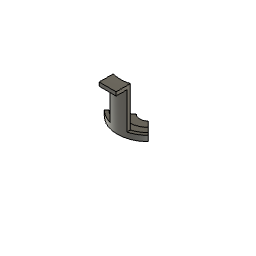
Wafer Loader 2 (Autodesk Fusion 360 design; units mm, degrees)
Autodesk Fusion 360 part; units mm, degrees
sketch "Sketch1" plane through (0, 0, 0) normal (0, 0, 1) x (1, 0, 0)
  circle A0 centre (0, 0) radius 51.3
  circle A1 centre (0, 0) radius 76
  circle A2 centre (0, 0) radius 23.25
  line L0 (0, 0) -> (-54.6679, -54.6679)
  line L1 (0, 0) -> (75, 0) construction
  line L2 (0, 0) -> (0, -76)
  line L3 (0, 0) -> (54.6679, -54.6679)
  line L4 (0, 0) -> (-23.1763, -71.3292)
  line L5 (0, 0) -> (75, 0) construction
  line L6 (0, 0) -> (23.1763, -71.3292)
  line L7 (-23.1763, -71.3292) -> (23.1763, -71.3292)
  line L8 (-23.1763, -71.3292) -> (-23.1763, -81.3292)
  line L9 (23.1763, -71.3292) -> (23.1763, -81.3292)
  line L10 (-23.1763, -81.3292) -> (23.1763, -81.3292)
  line L11 (-23.1763, -81.3292) -> (-23.1763, -111.3292)
  line L12 (23.1763, -81.3292) -> (23.1763, -111.3292)
  line L13 (-23.1763, -111.3292) -> (23.1763, -111.3292)
  circle A3 centre (0, 0) radius 85
  line L14 (-53.7401, -53.7401) -> (-60.1041, -60.1041)
  line L15 (53.7401, -53.7401) -> (60.1041, -60.1041)
  line L16 (-23.1763, -111.3292) -> (-23.1763, -101.3292)
  line L17 (-23.1763, -101.3292) -> (23.1763, -101.3292)
  dimension "d1" = 102.6
  dimension "d2" = 152
  dimension "d3" = 46.5
  dimension "d4" = 135
  dimension "d5" = 108
  dimension "d6" = 10
  dimension "d7" = 30
  dimension "d12" = 170
  dimension "d15" = 10
  constraint coincident A0.centre A1.centre
  constraint concentric A0 A1
  constraint horizontal L1
  constraint coincident A1 L2.end
  constraint vertical L2
  constraint symmetric A0.centre L2 A1.centre
  constraint symmetric L0.end L2 L3.end
  constraint horizontal L5
  constraint symmetric L2 A0.centre A1.centre
  constraint symmetric L2 L4.end L6.end
  constraint perpendicular L7 L8
  constraint symmetric L2 L8.end L9.end
  constraint perpendicular L10 L11
  constraint symmetric L2 L11.end L12.end
  constraint concentric A1 A3
  constraint coincident A1 L14.start
  constraint coincident L0 L14.start
  constraint coincident A3 L14.end
  constraint parallel L0 L14
  constraint coincident A1 L15.start
  constraint coincident L3 L15.start
  constraint coincident A3 L15.end
  constraint parallel L3 L15
  constraint perpendicular L13 L16
  constraint coincident L12 L17.end
  constraint perpendicular L12 L17
  measures "d1" diameter of A0
  measures "d2" diameter of A1
  measures "d3" diameter of A2
  measures "d4" angle of L0 L1
  measures "d5" angle of L4 L5
  measures "d6" distance of L4.end L8.end
  measures "d7" distance of L8.end L11.end
  measures "d12" diameter of A3
  measures "d15" distance of L11.end L16.end
extrude "Extrude1" add sketch "Sketch1" along normal blind 5 contours A0 A2 L0 L4 | A0 A1 L0 L4 L8 | A0 A1 L3 L6 L9 | A0 A2 L3 L6 | A0 A2 L2 L4 | A0 L2 L4 L7 | A0 L2 L6 L7 | A0 A2 L2 L6 | A1 L2 L7 L8 | A1 L2 L7 L9
extrude "Extrude2" add sketch "Sketch1" along normal blind 10 contours A0 A1 L0 L4 L8 | A0 A1 L3 L6 L9 | A0 L2 L4 L7 | A0 L2 L6 L7 | A1 L2 L7 L8 | A1 L2 L7 L9
extrude "Extrude3" add sketch "Sketch1" along normal blind 15 contours A1 L0 L3 A3 L14 L15 | A1 L0 L8 L11 A3 L14 | A1 L3 L9 L12 A3 L15 | A1 L8 L9 L10 | L10 L11 L12 A3
extrude "Extrude4" add sketch "Sketch1" along normal blind 15 contours L10 L11 L12 A3 | L11 L12 A3 L17 | L11 L12 L13 L16 L17
revolve "Revolve1" add 1 faces at (47.9183, -47.9183, 5) angle 45 about axis through (0, 0, -221.3292) along (0, 0, 1)
revolve "Revolve2" add 1 faces at (-47.9183, -47.9183, 5) angle 45 about axis through (0, 0, -221.3292) along (0, 0, -1)
extrude "Extrude5" cut sketch "Sketch1" along normal blind 15 contours L11 L12 L13 L16 L17
extrude "Extrude6" cut sketch "Sketch1" along normal blind 10 contours A1 L8 L9 L10 | L10 L11 L12 A3 | L11 L12 A3 L17
extrude "Extrude7" add 1 faces at (0, -92.8862, 10) along direction (0, 0, -1) blind 10
extrude "Extrude8" cut sketch "Sketch1" along normal blind 15 contours A0 A2 L0 L3 | A0 A1 L0 L3 | A1 L0 L3 A3 L14 L15
extrude "Extrude9" add sketch "Sketch1" along normal blind 100 contours A1 L8 L9 L10
extrude "Extrude10" cut sketch "Sketch1" along normal blind 100 contours L10 L11 L12 A3 | L11 L12 A3 L17
extrude "Extrude11" add sketch "Sketch1" along normal blind 100 contours L10 L11 L12 A3 | L11 L12 A3 L17 | L11 L12 L13 L16 L17
extrude "Extrude12" cut sketch "Sketch1" along normal blind 92 contours L10 L11 L12 A3 | L11 L12 A3 L17 | L11 L12 L13 L16 L17
extrude "Extrude13" add sketch "Sketch1" along normal blind 92 contours L10 L11 L12 A3
extrude "Extrude14" cut sketch "Sketch1" along normal blind 100 contours L11 L12 A3 L17 | L11 L12 L13 L16 L17
extrude "Extrude15" add 1 faces at (-5.4689, -81.6817, 100) along direction (0, 0, 1) blind 25
extrude "Extrude16" add sketch "Sketch1" along normal blind 125 contours L11 L12 A3 L17 | L11 L12 L13 L16 L17
extrude "Extrude17" cut sketch "Sketch1" along normal blind 115 contours L11 L12 A3 L17 | L11 L12 L13 L16 L17
